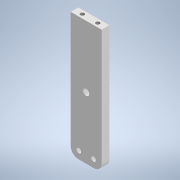
# Autodesk Inventor part: Z-Endstophalter2
Saved by Autodesk Inventor 2021.3 (Build 253353000, 353)
## iProperties
Created: 2021-04-27
Part Number: Z-Endstophalter2
Material: Generic
Document SubType Name: Modeling
Designer: Fabijan_Sven
Density: 1 g/cm^3
Appearance: Default
Author: Fabijan_Sven
Autodesk Inventor part; units mm, degrees
ref_plane "YZ Plane" through (0, 0, 0) normal (1, 0, 0) x (0, 1, 0)
ref_plane "XZ Plane" through (0, 0, 0) normal (0, 1, 0) x (-1, 0, 0)
ref_plane "XY Plane" through (0, 0, 0) normal (0, 0, 1) x (1, 0, 0)
sketch "Sketch1" plane through (0, 0, 0) normal (0, 0, 1) x (1, 0, 0)
  line L0 (40, 0) -> (60, 0)
  line L1 (60, 0) -> (60, -80)
  line L2 (60, -80) -> (40, -80)
  line L3 (40, -80) -> (40, 0)
  point P0 (0, 0)
  dimension "d0" = 40
  dimension "d1" = 20
  dimension "d2" = 80
  constraints: 8 end point, 2 parallel, 1 horizontal, 1 perpendicular, 1 point on line
  measures "d0" distance from line of L3 point (0, 0)
  measures "d1" distance of L1.end L2.end
  measures "d2" distance of L0.end L1.end
extrude "Extrusion1" add sketch "Sketch1" along normal blind 5
sketch "Sketch2" plane through (0, 0, 5) normal (0, 0, 1) x (1, 0, 0)
  circle A0 centre (45.25, -75) radius 1.5
  circle A1 centre (54.75, -75) radius 1.5
  line L0 (40, -80) -> (60, -80) projected
  line L1 (60, -80) -> (60, 0) projected
  point P0 (0, 0)
  dimension "d5" = 9.5
  dimension "d6" = 5
  dimension "d7" = 5
  dimension "d8" = 5.25
  dimension "d9" = 3
  dimension "d10" = 3
  constraints: 2 centre point
  measures "d5" distance of A1.centre A0.centre
  measures "d6" distance from line of L0 A1.centre
  measures "d7" distance from line of L0 A0.centre
  measures "d8" distance from line of L1 A1.centre
  measures "d9" diameter of A1
  measures "d10" diameter of A0
hole "Hole1" at (45.25, -75, 5) at (54.75, -75, 5) direction (0, 0, -1) diameter 3 depth 20 tip angle 118
fillet "Fillet1" radius 5 2 edges at (40, -80, 2.5) (60, -80, 2.5)
sketch "Sketch4" plane through (0, 0, 5) normal (0, 0, 1) x (1, 0, 0)
  circle A0 centre (50, -40) radius 2
  line L0 (40, 0) -> (40, -75) projected
  line L1 (60, 0) -> (40, 0) projected
  line L2 (45, -80) -> (55, -80) projected
  point P0 (0, 0)
  point P1 (40, -73.521)
  dimension "d32" = 4
  dimension "d33" = 10
  dimension "d34" = 40
  dimension "d42" = 80
  constraints: 1 centre point
  measures "d32" diameter of A0
  measures "d33" distance from line of A0.centre L0
  measures "d34" distance from line of L1 A0.centre
  measures "d42" distance between parallel lines of L2 L1
hole "Hole3" at (50, -40, 5) direction (0, 0, -1) diameter 4 depth 20 tip angle 118
sketch "Sketch6" plane through (40, 0, 0) normal (0, 1, 0) x (1, 0, 0)
  line L0 (5, 0) -> (5, -5) projected
  circle A0 centre (5, -2.5) radius 1.5
  line L1 (15, -5) -> (15, 0) projected
  circle A1 centre (15, -2.5) radius 1.5513
  point P0 (-40, 0)
  dimension "d50" = 3.1027
  dimension "d51" = 3
  constraints: 2 centre point, 2 midpoint
  measures "d50" diameter of A1
  measures "d51" diameter of A0
hole "Hole5" at (45, 0, 2.5) at (55, 0, 2.5) direction (0, -1, 0) diameter 2.459 depth 30 tip angle 118 thread size "M3x0.5" class "6H" standard "ISO Metric profile"
equation "\"d11\" = d9"
equation "\"d34\" = 0.5 * d42"
equation "\"d35\" = d32"
body "Solid1"
